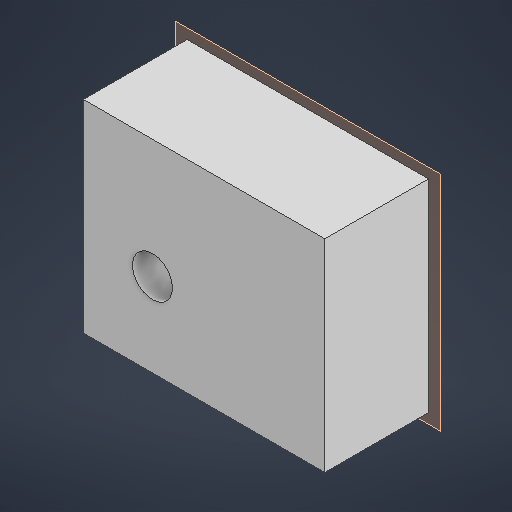
# Autodesk Inventor part: testdelete
Saved by Autodesk Inventor 2025.2 (Build 292293000, 293)
## iProperties
Created: 2025-06-16
Part Number: testdelete
Material: Generic
Document SubType Name: Modeling
Designer: Tiago
Density: 1 g/cm^3
Appearance: Default
Author: Tiago
Autodesk Inventor part; units mm, degrees
ref_plane "YZ Plane" through (0, 0, 0) normal (1, 0, 0) x (0, 1, 0)
ref_plane "XZ Plane" through (0, 0, 0) normal (0, 1, 0) x (-1, 0, 0)
sketch "Sketch1" plane through (0, 0, 0) normal (0, 0, 1) x (1, 0, 0)
  line L0 (0, 0) -> (9.3116, 0)
  line L1 (9.3116, 0) -> (9.3116, 7.8058)
  line L2 (9.3116, 7.8058) -> (0, 7.8058)
  line L3 (0, 7.8058) -> (0, 0)
  circle A0 centre (2.6618, 3.222) radius 0.7712
  dimension "d0" = 9.3116
  dimension "d1" = 7.8058
  dimension "d2" = 2.6618
  dimension "d3" = 3.222
  dimension "d4" = 1.5424
  constraints: 8 end point, 2 parallel, 1 centre point, 1 horizontal, 1 perpendicular
  measures "d0" distance between parallel lines of L3 L1
  measures "d1" distance between parallel lines of L0 L2
  measures "d2" distance from line of L3 A0.centre
  measures "d3" distance from line of L0 A0.centre
  measures "d4" diameter of A0
extrude "Extrusion1" add sketch "Sketch1" along normal blind 4
body "Solid1"
